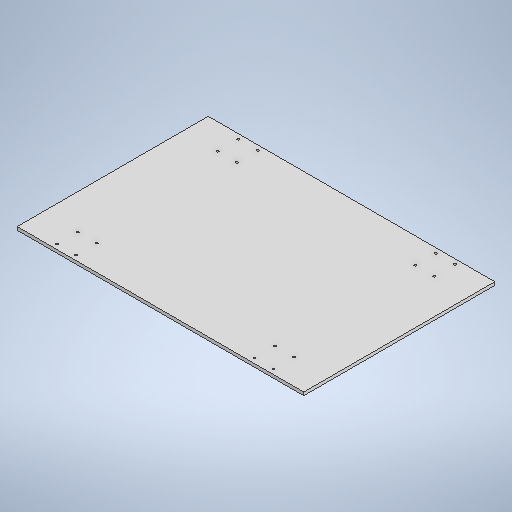
# Autodesk Inventor part: ChassisTest
Saved by Autodesk Inventor 2025.2 (Build 292293000, 293)
## iProperties
Created: 2025-01-16
Part Number: ChassisTest
Material: Generic
Document SubType Name: Modeling
Designer: Matt Tidd
Density: 1 g/cm^3
Appearance: Default
Author: Matt Tidd
Autodesk Inventor part; units mm, degrees
ref_plane "YZ Plane" through (0, 0, 0) normal (1, 0, 0) x (0, 1, 0)
ref_plane "XZ Plane" through (0, 0, 0) normal (0, 1, 0) x (-1, 0, 0)
ref_plane "XY Plane" through (0, 0, 0) normal (0, 0, 1) x (1, 0, 0)
sketch "Sketch1" plane through (0, 0, 0) normal (0, 1, 0) x (-1, 0, 0)
  line L0 (0, 0) -> (450, 0)
  line L1 (450, 0) -> (450, -300)
  line L2 (450, -300) -> (0, -300)
  line L3 (0, -300) -> (0, 0)
  dimension "d0" = 450
  dimension "d1" = 300
  constraints: 8 end point, 2 parallel, 1 horizontal, 1 perpendicular
  measures "d0" distance of L1.end L2.end
  measures "d1" distance of L0.end L1.end
extrude "Extrusion1" add sketch "Sketch1" along normal blind 5
sketch "Sketch2" plane through (0, 5, 0) normal (0, 1, 0) x (1, 0, 0)
  circle A0 centre (-55, 7.5) radius 1.75
  circle A1 centre (-55, 40) radius 1.75
  circle A2 centre (-85, 7.5) radius 1.75
  circle A3 centre (-85, 40) radius 1.75
  line L0 (0, 104.657) -> (0, 226.0583) construction
  line L1 (0, 0) -> (0, 300) construction
  circle A4 centre (-55, 260) radius 1.75
  circle A5 centre (-55, 292.5) radius 1.75
  circle A6 centre (-85, 260) radius 1.75
  circle A7 centre (-85, 292.5) radius 1.75
  line L2 (-450, 0) -> (0, 0) construction
  line L3 (-77.4228, 0) -> (-201.8841, 0) construction
  circle A8 centre (-365, 260) radius 1.75
  circle A9 centre (-365, 292.5) radius 1.75
  circle A10 centre (-395, 260) radius 1.75
  circle A11 centre (-395, 292.5) radius 1.75
  circle A12 centre (-365, 7.5) radius 1.75
  circle A13 centre (-365, 40) radius 1.75
  circle A14 centre (-395, 7.5) radius 1.75
  circle A15 centre (-395, 40) radius 1.75
  point P0 (-387.4228, 0)
  dimension "d5" = 3.5
  dimension "d7" = 3.5
  dimension "d8" = 3.5
  dimension "d9" = 3.5
  dimension "d12" = 252.5
  dimension "d19" = 310
  constraints: 16 centre point, 4 end point, 3 point on line, 1 horizontal, 1 vertical, 25 other
  measures "d5" diameter of A0
  measures "d7" diameter of A1
  measures "d8" diameter of A2
  measures "d9" diameter of A3
  measures "d12" distance of A0.centre A4.centre
  measures "d19" distance of A4.centre A8.centre
extrude "Extrusion2" cut sketch "Sketch2" against normal blind 310
equation "\"d24\" = d19"
body "Solid1"
